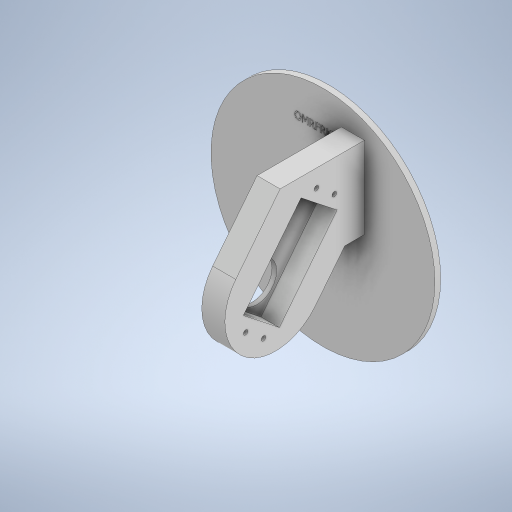
# Autodesk Inventor part: B
Saved by Autodesk Inventor 2023.2 (Build 272271000, 271)
## iProperties
Created: 2022-12-18
Part Number: B
Material: Generic
Document SubType Name: Modeling
Designer: omrfrkmll
Density: 1 g/cm^3
Appearance: Default
Author: omrfrkmll
Autodesk Inventor part; units mm, degrees
ref_plane "XZ Plane" through (0, 0, 0) normal (0, 1, 0) x (-1, 0, 0)
ref_plane "XY Plane" through (0, 0, 0) normal (0, 0, 1) x (1, 0, 0)
sketch "Sketch1" plane through (0, 0, 0) normal (0, 0, 1) x (1, 0, 0)
  circle A0 centre (0, 0) radius 48.5
  dimension "d0" = 97
  constraints: 1 centre point, 1 coincident
  measures "d0" diameter of A0
extrude "Extrusion1" add sketch "Sketch1" along normal blind 2.5
sketch "Sketch2" plane through (0, 0, 2.5) normal (0, 0, 1) x (1, 0, 0)
  line L0 (-8.1522, 0) -> (10.6782, 0)
  point P0 (0, 0)
  point P1 (0, 7.5)
  point P2 (0, -7.5)
  dimension "d3" = 15
  constraints: 2 end point, 1 horizontal, 1 point on line, 1 symmetric about line
  measures "d3" distance of point (0, -7.5) point (0, 7.5)
hole "Hole1" at (0, 7.5, 2.5) at (0, -7.5, 2.5) direction (0, 0, -1) diameter 2.1 depth 2.5
sketch "Sketch3" plane through (0, 0, 0) normal (0, 0, -1) x (-1, 0, 0)
  point P0 (0, 0)
  point P1 (0, 0)
  constraints: 1 coincident
hole "Hole2" at (0, 0, 0) direction (0, 0, 1) diameter 8 depth 2.5
sketch "Sketch4" plane through (0, 0, 2.5) normal (0, 0, 1) x (1, 0, 0)
  line L0 (-12.2991, 34.3731) -> (27.5625, 34.3731) construction
  line L1 (27.5625, 34.3731) -> (27.5625, 18.4619) construction
  line L2 (27.5625, 18.4619) -> (-12.2991, 18.4619) construction
  line L3 (-12.2991, 18.4619) -> (-12.2991, 34.3731) construction
  spline S0 degree 2 poles (-9.834, 33.9606) (-9.6611, 33.758) (-9.4685, 33.1652) (-9.4685, 32.7849) knots 0 0 0 1 2 2 2
  spline S1 degree 2 poles (-9.4685, 32.7849) (-9.4685, 32.4144) (-9.6562, 31.8141) (-9.834, 31.6116) knots 0 0 0 1 2 2 2
  spline S2 degree 2 poles (-9.834, 31.6116) (-10.0217, 31.3992) (-10.5182, 31.1966) (-10.8171, 31.1966) knots 0 0 0 1 2 2 2
  spline S3 degree 2 poles (-10.8171, 31.1966) (-11.1258, 31.1966) (-11.6198, 31.4066) (-11.8002, 31.6116) knots 0 0 0 1 2 2 2
  spline S4 degree 2 poles (-11.8002, 31.6116) (-11.9755, 31.8141) (-12.1633, 32.4094) (-12.1633, 32.7849) knots 0 0 0 1 2 2 2
  spline S5 degree 2 poles (-12.1633, 32.7849) (-12.1633, 33.1677) (-11.9731, 33.7506) (-11.7977, 33.9606) knots 0 0 0 1 2 2 2
  spline S6 degree 2 poles (-11.7977, 33.9606) (-11.6198, 34.1631) (-11.1234, 34.3731) (-10.8171, 34.3731) knots 0 0 0 1 2 2 2
  spline S7 degree 2 poles (-10.8171, 34.3731) (-10.5059, 34.3731) (-10.0069, 34.1557) (-9.834, 33.9606) knots 0 0 0 1 2 2 2
  spline S8 degree 2 poles (-9.8908, 32.7849) (-9.8908, 33.0862) (-10.0217, 33.553) (-10.1403, 33.7062) knots 0 0 0 1 2 2 2
  spline S9 degree 2 poles (-10.1403, 33.7062) (-10.2613, 33.8643) (-10.6022, 34.0223) (-10.8146, 34.0223) knots 0 0 0 1 2 2 2
  spline S10 degree 2 poles (-10.8146, 34.0223) (-11.0345, 34.0223) (-11.3654, 33.8692) (-11.4914, 33.7062) knots 0 0 0 1 2 2 2
  spline S11 degree 2 poles (-11.4914, 33.7062) (-11.6124, 33.5506) (-11.7409, 33.0813) (-11.7409, 32.7849) knots 0 0 0 1 2 2 2
  spline S12 degree 2 poles (-11.7409, 32.7849) (-11.7409, 32.1846) (-11.237, 31.5474) (-10.8146, 31.5474) knots 0 0 0 1 2 2 2
  spline S13 degree 2 poles (-10.8146, 31.5474) (-10.3923, 31.5474) (-9.8908, 32.1846) (-9.8908, 32.7849) knots 0 0 0 1 2 2 2
  line L4 (-6.4106, 31.2609) -> (-6.8157, 31.2609)
  line L5 (-6.8157, 31.2609) -> (-6.8157, 33.8865)
  line L6 (-6.8157, 33.8865) -> (-7.611, 32.1007)
  line L7 (-7.611, 32.1007) -> (-7.858, 32.1007)
  line L8 (-7.858, 32.1007) -> (-8.6459, 33.8865)
  line L9 (-8.6459, 33.8865) -> (-8.6459, 31.2609)
  line L10 (-8.6459, 31.2609) -> (-9.0239, 31.2609)
  line L11 (-9.0239, 31.2609) -> (-9.0239, 34.3089)
  line L12 (-9.0239, 34.3089) -> (-8.4706, 34.3089)
  line L13 (-8.4706, 34.3089) -> (-7.7098, 32.612)
  line L14 (-7.7098, 32.612) -> (-6.9737, 34.3089)
  line L15 (-6.9737, 34.3089) -> (-6.4106, 34.3089)
  line L16 (-6.4106, 34.3089) -> (-6.4106, 31.2609)
  line L17 (-3.4342, 31.2609) -> (-3.9603, 31.2609)
  line L18 (-3.9603, 31.2609) -> (-4.9236, 32.4736)
  line L19 (-4.9236, 32.4736) -> (-5.388, 32.4736)
  line L20 (-5.388, 32.4736) -> (-5.388, 31.2609)
  line L21 (-5.388, 31.2609) -> (-5.7931, 31.2609)
  line L22 (-5.7931, 31.2609) -> (-5.7931, 34.3089)
  line L23 (-5.7931, 34.3089) -> (-5.0076, 34.3089)
  spline S14 degree 2 poles (-5.0076, 34.3089) (-4.7458, 34.3089) (-4.3926, 34.252) (-4.232, 34.1483) knots 0 0 0 1 2 2 2
  spline S15 degree 2 poles (-4.232, 34.1483) (-4.0715, 34.0446) (-3.8862, 33.721) (-3.8862, 33.4814) knots 0 0 0 1 2 2 2
  spline S16 degree 2 poles (-3.8862, 33.4814) (-3.8862, 33.148) (-4.2271, 32.6959) (-4.5186, 32.5873) knots 0 0 0 1 2 2 2
  line L24 (-4.5186, 32.5873) -> (-3.4342, 31.2609)
  spline S17 degree 2 poles (-4.3086, 33.4493) (-4.3086, 33.5827) (-4.4025, 33.7877) (-4.5013, 33.8544) knots 0 0 0 1 2 2 2
  spline S18 degree 2 poles (-4.5013, 33.8544) (-4.5877, 33.9112) (-4.8174, 33.9581) (-4.9854, 33.9581) knots 0 0 0 1 2 2 2
  line L25 (-4.9854, 33.9581) -> (-5.388, 33.9581)
  line L26 (-5.388, 33.9581) -> (-5.388, 32.812)
  line L27 (-5.388, 32.812) -> (-5.0323, 32.812)
  spline S19 degree 2 poles (-5.0323, 32.812) (-4.8569, 32.812) (-4.5778, 32.8738) (-4.4815, 32.9701) knots 0 0 0 1 2 2 2
  spline S20 degree 2 poles (-4.4815, 32.9701) (-4.3926, 33.0541) (-4.3086, 33.2912) (-4.3086, 33.4493) knots 0 0 0 1 2 2 2
  line L28 (-1.3693, 33.9482) -> (-2.7871, 33.9482)
  line L29 (-2.7871, 33.9482) -> (-2.7871, 33.0887)
  line L30 (-2.7871, 33.0887) -> (-1.4286, 33.0887)
  line L31 (-1.4286, 33.0887) -> (-1.4286, 32.728)
  line L32 (-1.4286, 32.728) -> (-2.7871, 32.728)
  line L33 (-2.7871, 32.728) -> (-2.7871, 31.2609)
  line L34 (-2.7871, 31.2609) -> (-3.1922, 31.2609)
  line L35 (-3.1922, 31.2609) -> (-3.1922, 34.3089)
  line L36 (-3.1922, 34.3089) -> (-1.3693, 34.3089)
  line L37 (-1.3693, 34.3089) -> (-1.3693, 33.9482)
  line L38 (1.3527, 31.2609) -> (0.8266, 31.2609)
  line L39 (0.8266, 31.2609) -> (-0.1367, 32.4736)
  line L40 (-0.1367, 32.4736) -> (-0.6011, 32.4736)
  line L41 (-0.6011, 32.4736) -> (-0.6011, 31.2609)
  line L42 (-0.6011, 31.2609) -> (-1.0062, 31.2609)
  line L43 (-1.0062, 31.2609) -> (-1.0062, 34.3089)
  line L44 (-1.0062, 34.3089) -> (-0.2207, 34.3089)
  spline S21 degree 2 poles (-0.2207, 34.3089) (0.0411, 34.3089) (0.3943, 34.252) (0.5549, 34.1483) knots 0 0 0 1 2 2 2
  spline S22 degree 2 poles (0.5549, 34.1483) (0.7154, 34.0446) (0.9007, 33.721) (0.9007, 33.4814) knots 0 0 0 1 2 2 2
  spline S23 degree 2 poles (0.9007, 33.4814) (0.9007, 33.148) (0.5598, 32.6959) (0.2683, 32.5873) knots 0 0 0 1 2 2 2
  line L45 (0.2683, 32.5873) -> (1.3527, 31.2609)
  spline S24 degree 2 poles (0.4783, 33.4493) (0.4783, 33.5827) (0.3844, 33.7877) (0.2856, 33.8544) knots 0 0 0 1 2 2 2
  spline S25 degree 2 poles (0.2856, 33.8544) (0.1992, 33.9112) (-0.0305, 33.9581) (-0.1985, 33.9581) knots 0 0 0 1 2 2 2
  line L46 (-0.1985, 33.9581) -> (-0.6011, 33.9581)
  line L47 (-0.6011, 33.9581) -> (-0.6011, 32.812)
  line L48 (-0.6011, 32.812) -> (-0.2454, 32.812)
  spline S26 degree 2 poles (-0.2454, 32.812) (-0.0701, 32.812) (0.2091, 32.8738) (0.3054, 32.9701) knots 0 0 0 1 2 2 2
  spline S27 degree 2 poles (0.3054, 32.9701) (0.3943, 33.0541) (0.4783, 33.2912) (0.4783, 33.4493) knots 0 0 0 1 2 2 2
  line L49 (3.8178, 31.2609) -> (3.2916, 31.2609)
  line L50 (3.2916, 31.2609) -> (2.1777, 32.6786)
  line L51 (2.1777, 32.6786) -> (1.9998, 32.4786)
  line L52 (1.9998, 32.4786) -> (1.9998, 31.2609)
  line L53 (1.9998, 31.2609) -> (1.5947, 31.2609)
  line L54 (1.5947, 31.2609) -> (1.5947, 34.3089)
  line L55 (1.5947, 34.3089) -> (1.9998, 34.3089)
  line L56 (1.9998, 34.3089) -> (1.9998, 32.9084)
  line L57 (1.9998, 32.9084) -> (3.2496, 34.3089)
  line L58 (3.2496, 34.3089) -> (3.7437, 34.3089)
  line L59 (3.7437, 34.3089) -> (2.4815, 32.9479)
  line L60 (2.4815, 32.9479) -> (3.8178, 31.2609)
  line L61 (6.6731, 31.2609) -> (6.268, 31.2609)
  line L62 (6.268, 31.2609) -> (6.268, 33.8865)
  line L63 (6.268, 33.8865) -> (5.4727, 32.1007)
  line L64 (5.4727, 32.1007) -> (5.2257, 32.1007)
  line L65 (5.2257, 32.1007) -> (4.4377, 33.8865)
  line L66 (4.4377, 33.8865) -> (4.4377, 31.2609)
  line L67 (4.4377, 31.2609) -> (4.0598, 31.2609)
  line L68 (4.0598, 31.2609) -> (4.0598, 34.3089)
  line L69 (4.0598, 34.3089) -> (4.6131, 34.3089)
  line L70 (4.6131, 34.3089) -> (5.3739, 32.612)
  line L71 (5.3739, 32.612) -> (6.1099, 34.3089)
  line L72 (6.1099, 34.3089) -> (6.6731, 34.3089)
  line L73 (6.6731, 34.3089) -> (6.6731, 31.2609)
  line L74 (9.0567, 31.2609) -> (7.2906, 31.2609)
  line L75 (7.2906, 31.2609) -> (7.2906, 34.3089)
  line L76 (7.2906, 34.3089) -> (7.6957, 34.3089)
  line L77 (7.6957, 34.3089) -> (7.6957, 31.6215)
  line L78 (7.6957, 31.6215) -> (9.0567, 31.6215)
  line L79 (9.0567, 31.6215) -> (9.0567, 31.2609)
  line L80 (11.1414, 31.2609) -> (9.3753, 31.2609)
  line L81 (9.3753, 31.2609) -> (9.3753, 34.3089)
  line L82 (9.3753, 34.3089) -> (9.7804, 34.3089)
  line L83 (9.7804, 34.3089) -> (9.7804, 31.6215)
  line L84 (9.7804, 31.6215) -> (11.1414, 31.6215)
  line L85 (11.1414, 31.6215) -> (11.1414, 31.2609)
  point P0 (0, 0)
  constraints: 2 other
emboss "Emboss1" sketch "Sketch4" operation cut depth 1 direction (0, 0, -1)
ref_plane "Work Plane1" through (8, 0, 0) normal (1, 0, 0) x (0, 1, 0)
sketch "Sketch5" plane through (8, 0, 0) normal (1, 0, 0) x (0, 1, 0)
  line L0 (0, -9.2185) -> (0, 69.143)
  circle A0 centre (0, 41.0454) radius 8.5
  line L1 (30.0579, 29.9671) -> (-1.5565, 54.9595)
  line L2 (-1.5565, 54.9595) -> (-13.8977, 39.3484)
  line L3 (-13.8977, 39.3484) -> (17.7167, 14.356)
  line L4 (17.7167, 14.356) -> (30.0579, 29.9671)
  line L5 (14.2507, 42.4633) -> (15.5634, 44.1239)
  line L6 (35.4315, 25.719) -> (23.0903, 10.1079)
  line L7 (-6.9302, 59.2076) -> (-19.2713, 43.5965)
  line L8 (0, 41.0454) -> (-9.4755, 48.5362)
  arc A1 (13.606, 58.2564) -> (-13.606, 23.8344) centre (0, 41.0454) ccw
  line L9 (48.5, 2.5) -> (-48.5, 2.5) projected
  line L10 (37.9315, 2.5) -> (37.9315, 39.026)
  line L11 (37.9315, 39.026) -> (13.606, 58.2564)
  line L12 (-13.606, 23.8344) -> (2.5715, 11.0455)
  line L13 (2.5715, 11.0455) -> (2.5715, 2.5)
  line L14 (-6.9302, 59.2076) -> (-7.8214, 61.5433)
  point P0 (0, 0)
  point P1 (-7.7271, 47.154)
  dimension "d21" = 19.9
  dimension "d22" = 40.3
  dimension "d23" = 9.85
  dimension "d24" = 17
  dimension "d25" = 54
  dimension "d26" = 2.5
  dimension "d27" = 2.5
  constraints: 28 end point, 10 point on line, 4 perpendicular, 3 parallel, 3 point on circle, 2 centre point, 2 midpoint, 2 tangent, 2 vertical, 1 coincident, 1 other
  measures "d21" distance between parallel lines of L1 L3
  measures "d22" distance between parallel lines of L2 L4
  measures "d23" distance from line of L2 L8.start
  measures "d24" diameter of A0
  measures "d25" distance between parallel lines of L6 L7
  measures "d26" distance of L7.start L14.end
  measures "d27" distance from line of L10 L6.start
extrude "Extrusion2" add sketch "Sketch5" along normal blind 10 contours L12 A1 L0 L1 L2 L3 | L0 L3 L4 L1 A1 L11 L10 L9 L13 L12 | L3 L2 L8 A0 L0 | L0 A0 L1 L4 L3 | L8 L2 L1 L0 A0
sketch "Sketch6" plane through (18, 0, 0) normal (1, 0, 0) x (0, 0, -1)
  line L0 (9.2185, 0) -> (-69.143, 0)
  circle A0 centre (-41.0454, 0) radius 8.5
  line L1 (-29.9671, 30.0579) -> (-54.9595, -1.5565)
  line L2 (-54.9595, -1.5565) -> (-39.3484, -13.8977)
  line L3 (-39.3484, -13.8977) -> (-14.356, 17.7167)
  line L4 (-14.356, 17.7167) -> (-29.9671, 30.0579)
  line L5 (-42.4633, 14.2507) -> (-44.1239, 15.5634)
  line L6 (-25.719, 35.4315) -> (-10.1079, 23.0903)
  line L7 (-59.2076, -6.9302) -> (-43.5965, -19.2713)
  line L8 (-41.0454, 0) -> (-48.5362, -9.4755)
  arc A1 (-58.2564, 13.606) -> (-23.8344, -13.606) centre (-41.0454, 0) ccw
  line L9 (-2.5, 48.5) -> (-2.5, -48.5)
  line L10 (-2.5, 37.9315) -> (-39.026, 37.9315)
  line L11 (-39.026, 37.9315) -> (-58.2564, 13.606)
  line L12 (-23.8344, -13.606) -> (-11.0455, 2.5715)
  line L13 (-11.0455, 2.5715) -> (-2.5, 2.5715)
  line L14 (-59.2076, -6.9302) -> (-61.5433, -7.8214)
  circle A2 centre (-41.0454, 0) radius 8.5 projected
  point P0 (0, 0)
  point P1 (0, 0)
  point P2 (-47.154, -7.7271)
  dimension "d30" = 19.9
  dimension "d31" = 40.3
  dimension "d32" = 9.85
  dimension "d33" = 17
  dimension "d34" = 54
  dimension "d35" = 2.5
  dimension "d36" = 2.5
  constraints: 30 end point, 10 point on line, 4 perpendicular, 3 parallel, 3 point on circle, 2 centre point, 2 coincident, 2 midpoint, 2 tangent, 1 other
  measures "d30" distance between parallel lines of L1 L3
  measures "d31" distance between parallel lines of L2 L4
  measures "d32" distance from line of L2 L8.start
  measures "d33" diameter of A0
  measures "d34" distance between parallel lines of L6 L7
  measures "d35" distance of L7.start L14.end
  measures "d36" distance from line of L10 L6.start
extrude "Extrusion3" cut sketch "Sketch6" against normal blind 8 contours A0 L0 L1 L4 L3 | L0 L3 L2 L8 A0 | A0 L8 L2 L1 L0
sketch "Sketch7" plane through (18, 0, 0) normal (1, 0, 0) x (0, 0, -1)
  line L0 (-14.356, 17.7167) -> (-39.3484, -13.8977) projected
  line L1 (-29.9671, 30.0579) -> (-14.356, 17.7167) projected
  line L2 (-29.9671, 30.0579) -> (-14.356, 17.7167) projected
  circle A0 centre (-41.0454, 0) radius 8.5 projected
  line L3 (-41.0454, 0) -> (-33.5089, 9.5334)
  line L4 (-54.9595, -1.5565) -> (-29.9671, 30.0579) projected
  point P0 (0, 0)
  point P1 (-23.3243, 30.3652)
  point P2 (-15.5964, 24.2576)
  point P3 (-53.9703, -8.4079)
  point P4 (-46.2432, -14.5165)
  point P5 (-26.8522, 1.9095)
  dimension "d39" = 49.422
  dimension "d40" = 9.85
  dimension "d48" = 15.419
  dimension "d49" = 35.158
  dimension "d50" = 35.158
  dimension "d51" = 9.85
  dimension "d52" = 15.419
  dimension "d54" = 9.85
  constraints: 2 end point, 1 midpoint, 1 parallel
  measures "d39" distance of point (-53.97, -8.408) point (-23.324, 30.365)
  measures "d40" distance of point (-46.243, -14.516) point (-53.97, -8.408)
  measures "d48" distance of L3.start point (-53.97, -8.408)
  measures "d49" distance of L3.start point (-23.324, 30.365)
  measures "d50" distance of L3.start point (-15.596, 24.258)
  measures "d51" distance of point (-15.596, 24.258) point (-23.324, 30.365)
  measures "d52" distance of L3.start point (-46.243, -14.516)
  measures "d54" diameter of point (-46.243, -14.516) L3
hole "Hole3" at (18, 30.3652, 23.3243) at (18, 24.2576, 15.5964) at (18, -8.4079, 53.9703) at (18, -14.5165, 46.2432) direction (-1, 0, 0) diameter 2 depth 7
sketch "Sketch8" plane through (18, 0, 0) normal (1, 0, 0) x (0, 0, -1)
  point P0 (0, 0)
body "Solid1"
